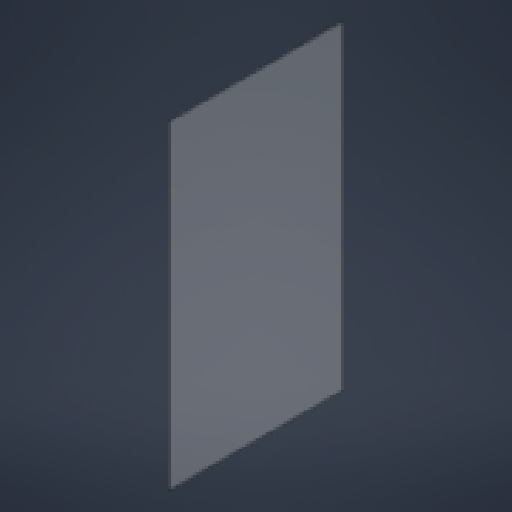
# Autodesk Inventor part: PLATE,HOPPER,BACK2
Saved by Autodesk Inventor 2026 (Build 300175000, 175)
## iProperties
Created: 2026-02-19
Part Number: PLATE,HOPPER,BACK2
Material: Polycarbonate, Clear
Document SubType Name: Sheet Metal
Designer: littl
Density: 1.2 g/cm^3
Sheet Metal Rule: Default
Appearance: Polycarbonate - Clear
Author: littl
Autodesk Inventor part; units mm, degrees
ref_plane "YZ Plane" through (0, 0, 0) normal (1, 0, 0) x (0, 1, 0)
ref_plane "XZ Plane" through (0, 0, 0) normal (0, 1, 0) x (-1, 0, 0)
ref_plane "XY Plane" through (0, 0, 0) normal (0, 0, 1) x (1, 0, 0)
sketch "Sketch1" plane through (0, 0, 0) normal (1, 0, 0) x (0, 1, 0)
  line L0 (0, 0) -> (-698.5, 0)
  line L1 (-698.5, 0) -> (-698.5, 381)
  line L2 (-698.5, 381) -> (0, 381)
  line L3 (0, 381) -> (0, 0)
  line L4 (-444.5, 381) -> (-444.5, 184.15)
  line L5 (-444.5, 184.15) -> (-698.5, 184.15)
  line L6 (-189.3272, 381) -> (-311.7065, 184.15)
  line L7 (-311.7065, 184.15) -> (-189.3272, 145.8189)
  line L8 (-189.3272, 145.8189) -> (-185.4527, 70.4)
  line L9 (-185.4527, 70.4) -> (-243.3711, 70.4)
  line L10 (-243.3711, 70.4) -> (-239.7544, 0)
  dimension "d0" = 698.5
  dimension "d1" = 381
  dimension "d3" = 254
  dimension "d4" = 196.85
  measures "d0" distance of L1.end L2.end
  measures "d1" distance of L0.end L1.end
  measures "d3" distance of L4.end L5.end
  measures "d4" distance of L4.start L4.end
extrude "Plate1" add sketch "Sketch1" along normal blind 3.175 contours L0 L1 L5 L4 L2 L6 L7 L8 L9 L10
equation "\"d2\" = Thickness"
equation "\"BendRadius\" = Thickness"
equation "\"BendReliefWidth\" = Thickness"
equation "\"BendReliefDepth\" = 0.5 * Thickness"
equation "\"CornerReliefSize\" = 4 * Thickness"
equation "\"MinimumRemnant\" = 2 * Thickness"
equation "\"TransitionRadius\" = BendRadius"
equation "\"JacobiRadiusSize\" = BendRadius"
equation "\"GapSize\" = Thickness"
equation "\"Thickness\" = 3.175"
body "Solid1"
